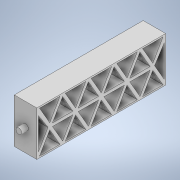
# Autodesk Inventor part: Arm support half scale
Saved by Autodesk Inventor 2020.2 (Build 242310000, 310)
## iProperties
Created: 2020-03-31
Part Number: Arm support half scale
Material: Generic
Document SubType Name: Modeling
Designer: Amaan Khalid
Density: 1 g/cm^3
Appearance: Default
Author: Amaan Khalid
Autodesk Inventor part; units mm, degrees
ref_plane "YZ Plane" through (0, 0, 0) normal (1, 0, 0) x (0, 1, 0)
ref_plane "XZ Plane" through (0, 0, 0) normal (0, 1, 0) x (-1, 0, 0)
ref_plane "XY Plane" through (0, 0, 0) normal (0, 0, 1) x (1, 0, 0)
sketch "Sketch1" plane through (0, 0, 0) normal (1, 0, 0) x (0, 1, 0)
  line L0 (23.7343, 15.4585) -> (23.7343, 4.0209)
  line L1 (23.7343, 4.0209) -> (33.6396, 9.7397)
  line L2 (33.6396, 9.7397) -> (23.7343, 15.4585)
  line L3 (32.268, 9.7397) -> (24.4201, 5.2087)
  line L4 (24.4201, 5.2087) -> (24.4201, 14.2706)
  line L5 (24.4201, 14.2706) -> (32.268, 9.7397)
  line L6 (33.6396, 9.7397) -> (23.7343, 4.0209)
  line L7 (33.6396, -1.698) -> (23.7343, 4.0209)
  line L8 (33.6396, 9.7397) -> (33.6396, -1.698)
  line L9 (32.9538, 8.5518) -> (25.1059, 4.0209)
  line L10 (25.1059, 4.0209) -> (32.9538, -0.5101)
  line L11 (32.9538, -0.5101) -> (32.9538, 8.5518)
  line L12 (23.7343, 4.0209) -> (23.7343, -7.4168)
  line L13 (23.7343, -7.4168) -> (33.6396, -1.698)
  line L14 (24.4201, -6.2289) -> (24.4201, 2.833)
  line L15 (24.4201, 2.833) -> (32.268, -1.698)
  line L16 (32.268, -1.698) -> (24.4201, -6.2289)
  line L17 (33.6396, -1.698) -> (33.6396, -13.1356)
  line L18 (33.6396, -13.1356) -> (23.7343, -7.4168)
  line L19 (32.9538, -11.9477) -> (32.9538, -2.8858)
  line L20 (25.1059, -7.4168) -> (32.9538, -11.9477)
  line L21 (32.9538, -2.8858) -> (25.1059, -7.4168)
  line L22 (23.7343, -7.4168) -> (23.7343, -18.8544)
  line L23 (24.4201, -17.6665) -> (24.4201, -8.6046)
  line L24 (23.7343, -18.8544) -> (33.6396, -13.1356)
  line L25 (32.268, -13.1356) -> (24.4201, -17.6665)
  line L26 (24.4201, -8.6046) -> (32.268, -13.1356)
  line L27 (33.6396, -13.1356) -> (33.6396, -24.5732)
  line L28 (32.9538, -14.3234) -> (25.1059, -18.8544)
  line L29 (25.1059, -18.8544) -> (32.9538, -23.3854)
  line L30 (33.6396, -24.5732) -> (23.7343, -18.8544)
  line L31 (32.9538, -23.3854) -> (32.9538, -14.3234)
  line L32 (23.7343, -18.8544) -> (23.7343, -30.292)
  line L33 (23.7343, -30.292) -> (33.6396, -24.5732)
  line L34 (32.268, -24.5732) -> (24.4201, -29.1042)
  line L35 (24.4201, -29.1042) -> (24.4201, -20.0422)
  line L36 (24.4201, -20.0422) -> (32.268, -24.5732)
  line L37 (23.7343, 4.0209) -> (13.8291, 9.7397)
  line L38 (13.8291, 9.7397) -> (23.7343, 15.4585)
  line L39 (15.2007, 9.7397) -> (23.0485, 5.2087)
  line L40 (23.0485, 5.2087) -> (23.0485, 14.2706)
  line L41 (23.0485, 14.2706) -> (15.2007, 9.7397)
  line L42 (23.7343, 4.0209) -> (13.8291, 9.7397)
  line L43 (13.8291, -1.698) -> (23.7343, 4.0209)
  line L44 (13.8291, 9.7397) -> (13.8291, -1.698)
  line L45 (14.5149, 8.5518) -> (22.3627, 4.0209)
  line L46 (22.3627, 4.0209) -> (14.5149, -0.5101)
  line L47 (14.5149, -0.5101) -> (14.5149, 8.5518)
  line L48 (13.8291, -1.698) -> (23.7343, 4.0209)
  line L49 (23.7343, -7.4168) -> (13.8291, -1.698)
  line L50 (23.0485, 2.833) -> (15.2007, -1.698)
  line L51 (23.0485, -6.2289) -> (23.0485, 2.833)
  line L52 (15.2007, -1.698) -> (23.0485, -6.2289)
  line L53 (13.8291, -13.1356) -> (23.7343, -7.4168)
  line L54 (15.2007, -13.1356) -> (23.0485, -17.6665)
  line L55 (23.0485, -17.6665) -> (23.0485, -8.6046)
  line L56 (23.7343, -18.8544) -> (13.8291, -13.1356)
  line L57 (23.0485, -8.6046) -> (15.2007, -13.1356)
  line L58 (23.7343, -7.4168) -> (13.8291, -1.698)
  line L59 (14.5149, -2.8858) -> (22.3627, -7.4168)
  line L60 (13.8291, -1.698) -> (13.8291, -13.1356)
  line L61 (14.5149, -11.9477) -> (14.5149, -2.8858)
  line L62 (13.8291, -13.1356) -> (23.7343, -7.4168)
  line L63 (22.3627, -7.4168) -> (14.5149, -11.9477)
  line L64 (13.8291, -24.5732) -> (23.7343, -18.8544)
  line L65 (23.0485, -29.1042) -> (23.0485, -20.0422)
  line L66 (23.7343, -30.292) -> (13.8291, -24.5732)
  line L67 (23.0485, -20.0422) -> (15.2007, -24.5732)
  line L68 (15.2007, -24.5732) -> (23.0485, -29.1042)
  line L69 (23.7343, -18.8544) -> (13.8291, -13.1356)
  line L70 (13.8291, -13.1356) -> (13.8291, -24.5732)
  line L71 (14.5149, -23.3854) -> (14.5149, -14.3234)
  line L72 (14.5149, -14.3234) -> (22.3627, -18.8544)
  line L73 (13.8291, -24.5732) -> (23.7343, -18.8544)
  line L74 (22.3627, -18.8544) -> (14.5149, -23.3854)
  line L75 (13.8291, 9.7397) -> (13.8291, 21.1773)
  line L76 (13.8291, 21.1773) -> (23.7343, 15.4585)
  line L77 (33.6396, 9.7397) -> (33.6396, 21.1773)
  line L78 (33.6396, 21.1773) -> (23.7343, 15.4585)
  line L79 (33.6396, 21.1773) -> (13.8291, 21.1773)
  line L80 (33.6396, -24.5732) -> (33.6396, -36.0108)
  line L81 (33.6396, -36.0108) -> (23.7343, -30.292)
  line L82 (13.8291, -24.5732) -> (13.8291, -36.0108)
  line L83 (13.8291, -36.0108) -> (23.7343, -30.292)
  line L84 (33.6396, -36.0108) -> (13.8291, -36.0108)
  line L85 (14.5149, 10.9275) -> (14.5149, 19.9894)
  line L86 (22.3627, 15.4585) -> (14.5149, 10.9275)
  line L87 (14.5149, 19.9894) -> (22.3627, 15.4585)
  line L88 (32.9538, 10.9275) -> (32.9538, 19.9894)
  line L89 (32.9538, 19.9894) -> (25.1059, 15.4585)
  line L90 (25.1059, 15.4585) -> (32.9538, 10.9275)
  line L91 (25.1059, -30.292) -> (32.9538, -34.823)
  line L92 (32.9538, -34.823) -> (32.9538, -25.761)
  line L93 (32.9538, -25.761) -> (25.1059, -30.292)
  line L94 (22.3627, -30.292) -> (14.5149, -34.823)
  line L95 (14.5149, -34.823) -> (14.5149, -25.761)
  line L96 (14.5149, -25.761) -> (22.3627, -30.292)
  line L97 (24.8388, 20.491) -> (30.3708, 20.491)
  line L98 (30.3708, 20.491) -> (23.7343, 16.2509)
  line L99 (23.7343, 16.2509) -> (16.3902, 20.491)
  line L100 (16.3902, 20.491) -> (24.8388, 20.491)
  line L101 (24.8388, -35.3246) -> (30.3708, -35.3246)
  line L102 (30.3708, -35.3246) -> (23.7343, -31.0844)
  line L103 (23.7343, -31.0844) -> (16.3902, -35.3246)
  line L104 (16.3902, -35.3246) -> (24.8388, -35.3246)
  dimension "d13" = 0.6858
  constraints: 210 end point, 61 symmetric about line, 5 vertical, 3 collinear, 2 point on line, 1 parallel, 2 other
  measures "d13" distance between parallel lines of L1 L3
extrude "Extrusion1" add sketch "Sketch1" along normal blind 10
sketch "Sketch2" plane through (0, 13.8291, 21.1773) normal (0, 0, 1) x (1, 0, 0)
  line L0 (0, 19.8105) -> (10, 19.8105) projected
  line L1 (10, 19.8105) -> (10, 9.9045)
  line L2 (10, 19.8105) -> (10, 0) projected
  line L3 (10, 9.9045) -> (4.9962, 9.9045)
  circle A0 centre (4.9962, 9.9045) radius 1.27
  point P0 (0, -13.8291)
  point P1 (0, 9.9053)
  dimension "d39" = 9.906
  dimension "d40" = 5.0038
  dimension "d41" = 2.54
  constraints: 4 end point, 1 centre point, 1 coincident, 1 perpendicular, 1 point on line
  measures "d39" distance of L0.end L1.end
  measures "d40" distance of L1.end L3.end
  measures "d41" diameter of A0
sketch "Sketch3" plane through (0, 13.8291, -36.0108) normal (0, 0, -1) x (-1, 0, 0)
  line L0 (0, 19.8105) -> (-10, 19.8105) projected
  line L1 (0, 10.5911) -> (-10, 10.5911) projected
  line L2 (0, 19.8105) -> (-10, 19.8105) projected
  line L3 (0, 19.8105) -> (0, 9.9045)
  line L4 (0, 0) -> (0, 19.8105) projected
  circle A0 centre (-5.0038, 9.9053) radius 1.27
  point P0 (0, -13.8291)
  dimension "d44" = 9.906
  dimension "d46" = 2.54
  constraints: 2 end point, 1 centre point, 1 point on line
  measures "d44" distance of L0.start L3.end
  measures "d46" diameter of A0
extrude "Extrusion4" add sketch "Sketch2" along normal blind 3
extrude "Extrusion5" add sketch "Sketch3" along normal blind 3
body "Solid1"
